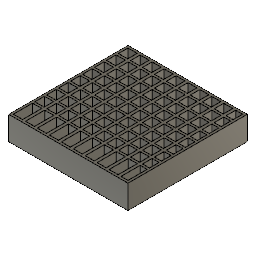
screw box v1 (Autodesk Fusion 360 design; units mm, degrees)
Autodesk Fusion 360 part; units mm, degrees
sketch "base" plane through (0, 0, 0) normal (0, 0, 1) x (1, 0, 0)
  line L0 (-63.5, 63.5) -> (63.5, 63.5)
  line L1 (63.5, 63.5) -> (63.5, -63.5)
  line L2 (63.5, -63.5) -> (-63.5, -63.5)
  line L3 (-63.5, -63.5) -> (-63.5, 63.5)
  line L4 (-63.5, 63.5) -> (63.5, -63.5) construction
  line L5 (63.5, 63.5) -> (-63.5, -63.5) construction
  dimension "d1" = 127
  dimension "d2" = 127
  constraint horizontal L0
  constraint perpendicular L0 L1
  constraint parallel L0 L2
  constraint parallel L1 L3
  constraint coincident L4 origin
  constraint coincident L5 origin
  measures "d1" distance of L0.start L0.end
  measures "d2" distance of L0.end L1.end
extrude "Extrude1" add sketch "base" along normal blind 25.4
shell "Shell1" thickness 2.54 removed faces 1 at (-21.1667, -21.1667, 25.4)
sketch "divider" plane through (0, 0, 2.54) normal (0, 0, 1) x (-1, 0, 0)
  line L0 (60.96, 60.96) -> (-60.96, 60.96)
  line L1 (-60.96, 60.96) -> (-60.96, -60.96)
  line L2 (-60.96, -60.96) -> (60.96, -60.96)
  line L3 (60.96, -60.96) -> (60.96, 60.96)
  line L4 (60.96, -50.8019) -> (-60.96, -50.8019)
  line L5 (-60.96, -50.8019) -> (-60.96, -48.3194)
  line L6 (-60.96, -48.3194) -> (60.96, -48.3194)
  line L7 (60.96, -48.3194) -> (60.96, -50.8019)
  line L8 (51.1232, -60.96) -> (48.0433, -60.96)
  line L9 (48.0433, -60.96) -> (48.0433, 60.96)
  line L10 (48.0433, 60.96) -> (51.1232, 60.96)
  line L11 (51.1232, 60.96) -> (51.1232, -60.96)
  line L12 (60.96, -35.6194) -> (60.96, -38.1019)
  line L13 (-60.96, -35.6194) -> (60.96, -35.6194)
  line L14 (60.96, -38.1019) -> (-60.96, -38.1019)
  line L15 (-60.96, -38.1019) -> (-60.96, -35.6194)
  line L16 (60.96, -22.9194) -> (60.96, -25.4019)
  line L17 (-60.96, -22.9194) -> (60.96, -22.9194)
  line L18 (60.96, -25.4019) -> (-60.96, -25.4019)
  line L19 (-60.96, -25.4019) -> (-60.96, -22.9194)
  line L20 (60.96, -10.2194) -> (60.96, -12.7019)
  line L21 (-60.96, -10.2194) -> (60.96, -10.2194)
  line L22 (60.96, -12.7019) -> (-60.96, -12.7019)
  line L23 (-60.96, -12.7019) -> (-60.96, -10.2194)
  line L24 (60.96, 2.4806) -> (60.96, -0.0019)
  line L25 (-60.96, 2.4806) -> (60.96, 2.4806)
  line L26 (60.96, -0.0019) -> (-60.96, -0.0019)
  line L27 (-60.96, -0.0019) -> (-60.96, 2.4806)
  line L28 (60.96, 15.1806) -> (60.96, 12.6981)
  line L29 (-60.96, 15.1806) -> (60.96, 15.1806)
  line L30 (60.96, 12.6981) -> (-60.96, 12.6981)
  line L31 (-60.96, 12.6981) -> (-60.96, 15.1806)
  line L32 (60.96, 27.8806) -> (60.96, 25.3981)
  line L33 (-60.96, 27.8806) -> (60.96, 27.8806)
  line L34 (60.96, 25.3981) -> (-60.96, 25.3981)
  line L35 (-60.96, 25.3981) -> (-60.96, 27.8806)
  line L36 (60.96, 40.5806) -> (60.96, 38.0981)
  line L37 (-60.96, 40.5806) -> (60.96, 40.5806)
  line L38 (60.96, 38.0981) -> (-60.96, 38.0981)
  line L39 (-60.96, 38.0981) -> (-60.96, 40.5806)
  line L40 (38.4232, -60.96) -> (35.3433, -60.96)
  line L41 (38.4232, 60.96) -> (38.4232, -60.96)
  line L42 (35.3433, -60.96) -> (35.3433, 60.96)
  line L43 (35.3433, 60.96) -> (38.4232, 60.96)
  line L44 (25.7232, -60.96) -> (22.6433, -60.96)
  line L45 (25.7232, 60.96) -> (25.7232, -60.96)
  line L46 (22.6433, -60.96) -> (22.6433, 60.96)
  line L47 (22.6433, 60.96) -> (25.7232, 60.96)
  line L48 (13.0232, -60.96) -> (9.9433, -60.96)
  line L49 (13.0232, 60.96) -> (13.0232, -60.96)
  line L50 (9.9433, -60.96) -> (9.9433, 60.96)
  line L51 (9.9433, 60.96) -> (13.0232, 60.96)
  line L52 (0.3232, -60.96) -> (-2.7567, -60.96)
  line L53 (0.3232, 60.96) -> (0.3232, -60.96)
  line L54 (-2.7567, -60.96) -> (-2.7567, 60.96)
  line L55 (-2.7567, 60.96) -> (0.3232, 60.96)
  line L56 (-12.3768, -60.96) -> (-15.4567, -60.96)
  line L57 (-12.3768, 60.96) -> (-12.3768, -60.96)
  line L58 (-15.4567, -60.96) -> (-15.4567, 60.96)
  line L59 (-15.4567, 60.96) -> (-12.3768, 60.96)
  line L60 (-25.0768, -60.96) -> (-28.1567, -60.96)
  line L61 (-25.0768, 60.96) -> (-25.0768, -60.96)
  line L62 (-28.1567, -60.96) -> (-28.1567, 60.96)
  line L63 (-28.1567, 60.96) -> (-25.0768, 60.96)
  line L64 (-37.7768, -60.96) -> (-40.8567, -60.96)
  line L65 (-37.7768, 60.96) -> (-37.7768, -60.96)
  line L66 (-40.8567, -60.96) -> (-40.8567, 60.96)
  line L67 (-40.8567, 60.96) -> (-37.7768, 60.96)
  line L68 (-50.4768, -60.96) -> (-53.5567, -60.96)
  line L69 (-50.4768, 60.96) -> (-50.4768, -60.96)
  line L70 (-53.5567, -60.96) -> (-53.5567, 60.96)
  line L71 (-53.5567, 60.96) -> (-50.4768, 60.96)
  dimension "d6" = 10.1581
  dimension "d7" = 9.8368
  dimension "d12" = 0
  dimension "d13" = 12.7
  dimension "d16" = -12.7
  dimension "d17" = 0
  constraint horizontal L4
  constraint vertical L5
  constraint horizontal L6
  constraint vertical L7
  constraint coincident L1 L5.end
  constraint coincident L3 L4.start
  constraint horizontal L8
  constraint vertical L9
  constraint horizontal L10
  constraint vertical L11
  constraint coincident L0 L9.end
  constraint coincident L2 L8.start
  measures "d6" distance of L2 L4
  measures "d7" distance of L3 L11
extrude "Extrude2" add sketch "divider" along normal blind 22.86 contours L0 L9 L10 L11 L37 | L3 L11 L36 L37 L38 | L9 L11 L37 L38 | L0 L37 L41 L42 L43 | L9 L37 L38 L41 | L9 L11 L33 L38 | L3 L11 L32 L33 L34 | L37 L38 L41 L42 | L9 L11 L33 L34 | L0 L37 L45 L46 L47 | L37 L38 L42 L45 | L33 L38 L41 L42 | L9 L33 L34 L41 | L9 L11 L29 L34 | L3 L11 L28 L29 L30 | L37 L38 L45 L46 | L33 L34 L41 L42 | L9 L11 L29 L30 | L0 L37 L49 L50 L51 | L37 L38 L46 L49 | L33 L38 L45 L46 | L33 L34 L42 L45 | L29 L34 L41 L42 | L9 L29 L30 L41 | L9 L11 L25 L30 | L3 L11 L24 L25 L26 | L37 L38 L49 L50 | L33 L34 L45 L46 | L29 L30 L41 L42 | L9 L11 L25 L26 | L0 L37 L53 L54 L55 | L37 L38 L50 L53 | L33 L38 L49 L50 | L33 L34 L46 L49 | L29 L34 L45 L46 | L29 L30 L42 L45 | L25 L30 L41 L42 | L9 L25 L26 L41 | L9 L11 L21 L26 | L3 L11 L20 L21 L22 | L37 L38 L53 L54 | L33 L34 L49 L50 | L29 L30 L45 L46 | L25 L26 L41 L42 | L9 L11 L21 L22 | L0 L37 L57 L58 L59 | L37 L38 L54 L57 | L33 L38 L53 L54 | L33 L34 L50 L53 | L29 L34 L49 L50 | L29 L30 L46 L49 | L25 L30 L45 L46 | L25 L26 L42 L45 | L21 L26 L41 L42 | L9 L21 L22 L41 | L9 L11 L17 L22 | L3 L11 L16 L17 L18 | L37 L38 L57 L58 | L33 L34 L53 L54 | L29 L30 L49 L50 | L25 L26 L45 L46 | L21 L22 L41 L42 | L9 L11 L17 L18 | L0 L37 L61 L62 L63 | L37 L38 L58 L61 | L33 L38 L57 L58 | L33 L34 L54 L57 | L29 L34 L53 L54 | L29 L30 L50 L53 | L25 L30 L49 L50 | L25 L26 L46 L49 | L21 L26 L45 L46 | L21 L22 L42 L45 | L17 L22 L41 L42 | L9 L17 L18 L41 | L9 L11 L13 L18 | L3 L11 L12 L13 L14 | L37 L38 L61 L62 | L33 L34 L57 L58 | L29 L30 L53 L54 | L25 L26 L49 L50 | L21 L22 L45 L46 | L17 L18 L41 L42 | L9 L11 L13 L14 | L0 L37 L65 L66 L67 | L37 L38 L62 L65 | L33 L38 L61 L62 | L33 L34 L58 L61 | L29 L34 L57 L58 | L29 L30 L54 L57 | L25 L30 L53 L54 | L25 L26 L50 L53 | L21 L26 L49 L50 | L21 L22 L46 L49 | L17 L22 L45 L46 | L17 L18 L42 L45 | L13 L18 L41 L42 | L9 L13 L14 L41 | L6 L9 L11 L14 | L3 L4 L6 L7 L11 | L37 L38 L65 L66 | L33 L34 L61 L62 | L29 L30 L57 L58 | L25 L26 L53 L54 | L21 L22 L49 L50 | L17 L18 L45 L46 | L13 L14 L41 L42 | L4 L6 L9 L11 | L0 L37 L69 L70 L71 | L37 L38 L66 L69 | L33 L38 L65 L66 | L33 L34 L62 L65 | L29 L34 L61 L62 | L29 L30 L58 L61 | L25 L30 L57 L58 | L25 L26 L54 L57 | L21 L26 L53 L54 | L21 L22 L50 L53 | L17 L22 L49 L50 | L17 L18 L46 L49 | L13 L18 L45 L46 | L13 L14 L42 L45 | L6 L14 L41 L42 | L4 L6 L9 L41 | L2 L4 L8 L9 L11 | L37 L38 L69 L70 | L33 L34 L65 L66 | L29 L30 L61 L62 | L25 L26 L57 L58 | L21 L22 L53 L54 | L17 L18 L49 L50 | L13 L14 L45 L46 | L4 L6 L41 L42 | L1 L37 L38 L39 L70 | L33 L38 L69 L70 | L33 L34 L66 L69 | L29 L34 L65 L66 | L29 L30 L62 L65 | L25 L30 L61 L62 | L25 L26 L58 L61 | L21 L26 L57 L58 | L21 L22 L54 L57 | L17 L22 L53 L54 | L17 L18 L50 L53 | L13 L18 L49 L50 | L13 L14 L46 L49 | L6 L14 L45 L46 | L4 L6 L42 L45 | L2 L4 L40 L41 L42 | L33 L34 L69 L70 | L29 L30 L65 L66 | L25 L26 L61 L62 | L21 L22 L57 L58 | L17 L18 L53 L54 | L13 L14 L49 L50 | L4 L6 L45 L46 | L1 L33 L34 L35 L70 | L29 L34 L69 L70 | L29 L30 L66 L69 | L25 L30 L65 L66 | L25 L26 L62 L65 | L21 L26 L61 L62 | L21 L22 L58 L61 | L17 L22 L57 L58 | L17 L18 L54 L57 | L13 L18 L53 L54 | L13 L14 L50 L53 | L6 L14 L49 L50 | L4 L6 L46 L49 | L2 L4 L44 L45 L46 | L29 L30 L69 L70 | L25 L26 L65 L66 | L21 L22 L61 L62 | L17 L18 L57 L58 | L13 L14 L53 L54 | L4 L6 L49 L50 | L1 L29 L30 L31 L70 | L25 L30 L69 L70 | L25 L26 L66 L69 | L21 L26 L65 L66 | L21 L22 L62 L65 | L17 L22 L61 L62 | L17 L18 L58 L61 | L13 L18 L57 L58 | L13 L14 L54 L57 | L6 L14 L53 L54 | L4 L6 L50 L53 | L2 L4 L48 L49 L50 | L25 L26 L69 L70 | L21 L22 L65 L66 | L17 L18 L61 L62 | L13 L14 L57 L58 | L4 L6 L53 L54 | L1 L25 L26 L27 L70 | L21 L26 L69 L70 | L21 L22 L66 L69 | L17 L22 L65 L66 | L17 L18 L62 L65 | L13 L18 L61 L62 | L13 L14 L58 L61 | L6 L14 L57 L58 | L4 L6 L54 L57 | L2 L4 L52 L53 L54 | L21 L22 L69 L70 | L17 L18 L65 L66 | L13 L14 L61 L62 | L4 L6 L57 L58 | L1 L21 L22 L23 L70 | L17 L22 L69 L70 | L17 L18 L66 L69 | L13 L18 L65 L66 | L13 L14 L62 L65 | L6 L14 L61 L62 | L4 L6 L58 L61 | L2 L4 L56 L57 L58 | L17 L18 L69 L70 | L13 L14 L65 L66 | L4 L6 L61 L62 | L1 L17 L18 L19 L70 | L13 L18 L69 L70 | L13 L14 L66 L69 | L6 L14 L65 L66 | L4 L6 L62 L65 | L2 L4 L60 L61 L62 | L13 L14 L69 L70 | L4 L6 L65 L66 | L1 L13 L14 L15 L70 | L6 L14 L69 L70 | L4 L6 L66 L69 | L2 L4 L64 L65 L66 | L4 L6 L69 L70 | L1 L4 L5 L6 L70 | L2 L4 L68 L69 L70
